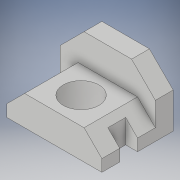
# Autodesk Inventor part: 410571040加分題
Saved by Autodesk Inventor 2017 (Build 210142000, 142)
## iProperties
Part Number: 410571040加分題
Material: 一般
Document SubType Name: Modeling
Designer: user
Density: 1 g/cm^3
Appearance: 預設
Author: user
Autodesk Inventor part; units mm, degrees
ref_plane "YZ Plane" through (0, 0, 0) normal (1, 0, 0) x (0, 1, 0)
ref_plane "XZ Plane" through (0, 0, 0) normal (0, 1, 0) x (-1, 0, 0)
ref_plane "XY Plane" through (0, 0, 0) normal (0, 0, 1) x (1, 0, 0)
sketch "草圖1" plane through (0, 0, 0) normal (0, 0, 1) x (1, 0, 0)
  line L0 (0, 0) -> (0, 8)
  line L1 (0, 8) -> (12, 20)
  line L2 (12, 20) -> (52, 20)
  line L3 (52, 20) -> (64, 8)
  line L4 (64, 8) -> (64, 0)
  line L5 (64, 0) -> (0, 0)
  dimension "d0" = 8
  dimension "d1" = 8
  dimension "d2" = 40
  dimension "d3" = 64
  dimension "d4" = 20
  dimension "d5" = 12
  constraints: 12 end point, 2 perpendicular, 1 parallel, 1 vertical
  measures "d0" distance of L0.start L0.end
  measures "d1" distance of L3.end L4.end
  measures "d2" distance of L1.end L2.end
  measures "d3" distance of L4.end L0.start
  measures "d4" distance between parallel lines of L5 L2
  measures "d5" horizontal distance of L1.end L0.end
extrude "擠出1" add sketch "草圖1" against normal blind 36
sketch "草圖3" plane through (12, 20, 0) normal (0, 1, 0) x (1, 0, 0)
  line L0 (52, 0) -> (52, 36) projected
  line L1 (52, 24) -> (44, 24)
  line L2 (44, 24) -> (44, 12)
  line L3 (44, 12) -> (52, 12)
  line L4 (40, 0) -> (52, 0) projected
  point P0 (-12, 0)
  dimension "d10" = 12
  dimension "d11" = 12
  dimension "d12" = 8
  constraints: 6 end point, 3 perpendicular, 2 point on line
  measures "d10" distance between parallel lines of L4 L3
  measures "d11" distance of L1.end L2.end
  measures "d12" distance of L1.start L1.end
extrude "擠出2" cut sketch "草圖3" against normal blind 48
sketch "草圖5" plane through (12, 20, 0) normal (0, 1, 0) x (1, 0, 0)
  line L0 (-12, 0) -> (-12, 36) projected
  line L1 (-12, 12) -> (-4, 12)
  line L2 (-4, 12) -> (-4, 24)
  line L3 (-4, 24) -> (-12, 24)
  line L4 (-12, 0) -> (0, 0) projected
  dimension "d18" = 12
  dimension "d19" = 12
  dimension "d20" = 8
  constraints: 6 end point, 2 perpendicular, 2 point on line, 1 horizontal
  measures "d18" distance between parallel lines of L1 L4
  measures "d19" distance of L1.end L2.end
  measures "d20" distance of L1.start L1.end
extrude "擠出3" cut sketch "草圖5" against normal blind 48
sketch "草圖6" plane through (12, 20, 0) normal (0, 1, 0) x (1, 0, 0)
  circle A0 centre (20, 18) radius 12
  line L0 (0, 0) -> (40, 0) projected
  line L1 (40, 0) -> (40, 36) projected
  point P0 (-12, 0)
  dimension "d23" = 24
  dimension "d24" = 18
  dimension "d25" = 20
  constraints: 1 centre point
  measures "d23" diameter of A0
  measures "d24" distance from line of A0.centre L0
  measures "d25" distance from line of A0.centre L1
extrude "擠出4" cut sketch "草圖6" against normal blind 48
sketch "草圖7" plane through (0, 0, -36) normal (0, 0, -1) x (-1, 0, 0)
  line L0 (-64, 0) -> (-64, 24)
  line L1 (-64, 24) -> (-48, 40)
  line L2 (-48, 40) -> (-16, 40)
  line L3 (-16, 40) -> (0, 24)
  line L4 (0, 0) -> (0, 8) projected
  line L5 (0, 24) -> (0, 8)
  line L6 (0, 8) -> (0, 0)
  line L7 (-64, 0) -> (0, 0) projected
  dimension "d28" = 32
  dimension "d29" = 16
  dimension "d30" = 40
  dimension "d31" = 16
  dimension "d32" = 16
  constraints: 12 end point, 1 collinear, 1 parallel, 1 perpendicular, 1 vertical
  measures "d28" distance of L1.end L2.end
  measures "d29" horizontal distance of L1.end L0.end
  measures "d30" distance between parallel lines of L7 L2
  measures "d31" horizontal distance of L3.end L2.end
  measures "d32" horizontal distance of L1.end L0.end
extrude "擠出5" add sketch "草圖7" along normal blind 12
